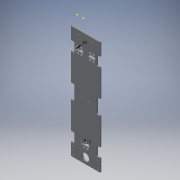
# Autodesk Inventor part: XCartFloor
Saved by Autodesk Inventor 2019 (Build 230136000, 136)
## iProperties
Created: 2019-08-19
Part Number: XCartFloor
Material: Generic
Document SubType Name: Modeling
Designer: Bruno
Density: 1 g/cm^3
Appearance: Default
Author: Bruno
Autodesk Inventor part; units mm, degrees
ref_plane "YZ Plane" through (0, 0, 0) normal (1, 0, 0) x (0, 1, 0)
ref_plane "XZ Plane" through (0, 0, 0) normal (0, 1, 0) x (-1, 0, 0)
ref_plane "XY Plane" through (0, 0, 0) normal (0, 0, 1) x (1, 0, 0)
sketch "Sketch1" plane through (0, 0, 0) normal (0, 0, 1) x (1, 0, 0)
  line L0 (100.0979, -38.5222) -> (0.0979, -38.5222)
  line L1 (0.0979, -426.5222) -> (100.0979, -426.5222)
  line L2 (82.7645, -93.1222) -> (58.7645, -93.1222)
  line L3 (58.7645, -93.1222) -> (58.7645, -101.9222)
  line L4 (58.7645, -101.9222) -> (82.7645, -101.9222)
  line L5 (82.7645, -101.9222) -> (82.7645, -93.1222)
  line L6 (41.4312, -93.1222) -> (17.4312, -93.1222)
  line L7 (17.4312, -93.1222) -> (17.4312, -101.9222)
  line L8 (17.4312, -101.9222) -> (41.4312, -101.9222)
  line L9 (41.4312, -101.9222) -> (41.4312, -93.1222)
  line L10 (38.0979, -363.1222) -> (62.0979, -363.1222)
  line L11 (62.0979, -363.1222) -> (62.0979, -371.9222)
  line L12 (62.0979, -371.9222) -> (38.0979, -371.9222)
  line L13 (38.0979, -371.9222) -> (38.0979, -363.1222)
  line L14 (173.8639, -93.5222) -> (-221.1361, -93.5222)
  line L15 (173.8639, -101.5222) -> (-221.1361, -101.5222)
  line L16 (173.8639, -371.5222) -> (-221.1361, -371.5222)
  line L17 (173.8639, -363.5222) -> (-221.1361, -363.5222)
  line L18 (34.8712, -93.1222) -> (34.8712, -93.5222) construction
  line L19 (34.8712, -101.5222) -> (34.8712, -101.9222) construction
  line L20 (58.7645, -93.1222) -> (41.4312, -93.1222) construction
  line L21 (10.9151, -363.1222) -> (10.9151, -363.5222) construction
  line L22 (10.9151, -371.5222) -> (10.9151, -371.9222) construction
  line L23 (38.0979, -363.1222) -> (12.0979, -363.1222) construction
  line L24 (62.0979, -363.1222) -> (88.0979, -363.1222) construction
  line L25 (0, 0) -> (0, -9.7735) construction
  circle A0 centre (65.5979, -390.5222) radius 1.625
  circle A1 centre (65.5979, -421.5222) radius 1.625
  circle A2 centre (34.5979, -421.5222) radius 1.625
  circle A3 centre (34.5979, -390.5222) radius 1.625
  line L26 (65.5979, -390.5222) -> (34.5979, -390.5222) construction
  line L27 (34.5979, -390.5222) -> (34.5979, -421.5222) construction
  line L28 (34.5979, -421.5222) -> (65.5979, -421.5222) construction
  line L29 (65.5979, -421.5222) -> (65.5979, -390.5222) construction
  circle A4 centre (50.0979, -406.0222) radius 12.5
  line L30 (50.0979, -390.5222) -> (50.0979, -406.0222) construction
  line L31 (50.0979, -406.0222) -> (65.5979, -406.0222) construction
  line L32 (72.2645, -85.1222) -> (80.2645, -85.1222)
  line L33 (80.2645, -85.1222) -> (80.2645, -89.1222)
  line L34 (80.2645, -89.1222) -> (72.2645, -89.1222)
  line L35 (72.2645, -89.1222) -> (72.2645, -85.1222)
  line L36 (80.2645, -89.1222) -> (82.7645, -89.1222) construction
  line L37 (82.7645, -89.1222) -> (82.7645, -93.1222) construction
  line L38 (69.2645, -85.1222) -> (61.2645, -85.1222)
  line L39 (61.2645, -85.1222) -> (61.2645, -89.1222)
  line L40 (61.2645, -89.1222) -> (69.2645, -89.1222)
  line L41 (69.2645, -89.1222) -> (69.2645, -85.1222)
  line L42 (58.7645, -93.1222) -> (58.7645, -89.1222) construction
  line L43 (58.7645, -89.1222) -> (61.2645, -89.1222) construction
  line L44 (72.2645, -105.9222) -> (80.2645, -105.9222)
  line L45 (80.2645, -105.9222) -> (80.2645, -109.9222)
  line L46 (80.2645, -109.9222) -> (72.2645, -109.9222)
  line L47 (72.2645, -109.9222) -> (72.2645, -105.9222)
  line L48 (80.2645, -105.9222) -> (80.2645, -101.9222) construction
  line L49 (69.2645, -105.9222) -> (61.2645, -105.9222)
  line L50 (61.2645, -105.9222) -> (61.2645, -109.9222)
  line L51 (61.2645, -109.9222) -> (69.2645, -109.9222)
  line L52 (69.2645, -109.9222) -> (69.2645, -105.9222)
  line L53 (38.9312, -85.1222) -> (30.9312, -85.1222)
  line L54 (30.9312, -85.1222) -> (30.9312, -89.1222)
  line L55 (30.9312, -89.1222) -> (38.9312, -89.1222)
  line L56 (38.9312, -89.1222) -> (38.9312, -85.1222)
  line L57 (27.9312, -85.1222) -> (19.9312, -85.1222)
  line L58 (19.9312, -85.1222) -> (19.9312, -89.1222)
  line L59 (19.9312, -89.1222) -> (27.9312, -89.1222)
  line L60 (27.9312, -89.1222) -> (27.9312, -85.1222)
  line L61 (30.9312, -105.9222) -> (38.9312, -105.9222)
  line L62 (38.9312, -105.9222) -> (38.9312, -109.9222)
  line L63 (38.9312, -109.9222) -> (30.9312, -109.9222)
  line L64 (30.9312, -109.9222) -> (30.9312, -105.9222)
  line L65 (27.9312, -105.9222) -> (19.9312, -105.9222)
  line L66 (19.9312, -105.9222) -> (19.9312, -109.9222)
  line L67 (19.9312, -109.9222) -> (27.9312, -109.9222)
  line L68 (27.9312, -109.9222) -> (27.9312, -105.9222)
  line L69 (41.4312, -93.1222) -> (41.4312, -89.1222) construction
  line L70 (41.4312, -89.1222) -> (38.9312, -89.1222) construction
  line L71 (17.4312, -93.1222) -> (17.4312, -89.1222) construction
  line L72 (17.4312, -89.1222) -> (19.9312, -89.1222) construction
  line L73 (51.5979, -355.1222) -> (59.5979, -355.1222)
  line L74 (59.5979, -355.1222) -> (59.5979, -359.1222)
  line L75 (59.5979, -359.1222) -> (51.5979, -359.1222)
  line L76 (51.5979, -359.1222) -> (51.5979, -355.1222)
  line L77 (48.5979, -355.1222) -> (40.5979, -355.1222)
  line L78 (40.5979, -355.1222) -> (40.5979, -359.1222)
  line L79 (40.5979, -359.1222) -> (48.5979, -359.1222)
  line L80 (48.5979, -359.1222) -> (48.5979, -355.1222)
  line L81 (51.5979, -375.9222) -> (59.5979, -375.9222)
  line L82 (59.5979, -375.9222) -> (59.5979, -379.9222)
  line L83 (59.5979, -379.9222) -> (51.5979, -379.9222)
  line L84 (51.5979, -379.9222) -> (51.5979, -375.9222)
  line L85 (48.5979, -375.9222) -> (40.5979, -375.9222)
  line L86 (40.5979, -375.9222) -> (40.5979, -379.9222)
  line L87 (40.5979, -379.9222) -> (48.5979, -379.9222)
  line L88 (48.5979, -379.9222) -> (48.5979, -375.9222)
  line L89 (59.5979, -359.1222) -> (62.0979, -359.1222) construction
  line L90 (62.0979, -359.1222) -> (62.0979, -363.1222) construction
  line L91 (38.0979, -363.1222) -> (38.0979, -359.1222) construction
  line L92 (38.0979, -359.1222) -> (40.5979, -359.1222) construction
  line L93 (59.5979, -375.9222) -> (59.5979, -371.9222) construction
  circle A5 centre (73.5979, -50.5222) radius 2.125
  circle A6 centre (26.5979, -50.5222) radius 2.125
  line L94 (73.5979, -50.5222) -> (100.0979, -50.5222) construction
  line L95 (26.5979, -50.5222) -> (0.0979, -50.5222) construction
  line L96 (96.5979, -57.5222) -> (88.5979, -57.5222) projected
  line L97 (11.5979, -57.5222) -> (3.5979, -57.5222) projected
  line L98 (8.0979, -43.5222) -> (8.0979, -57.5222) projected
  line L99 (7.0979, -57.5222) -> (7.0979, -43.5222) projected
  line L100 (93.0979, -43.5222) -> (93.0979, -57.5222) projected
  line L101 (92.0979, -57.5222) -> (92.0979, -43.5222) projected
  line L102 (7.5979, -57.5222) -> (7.5979, -426.5222) construction
  line L103 (92.5979, -57.5222) -> (92.5979, -426.5222) construction
  circle A7 centre (92.5979, -419.5222) radius 2.125
  circle A8 centre (92.5979, -392.5222) radius 2.125
  circle A9 centre (7.5979, -419.5222) radius 2.125
  circle A10 centre (7.5979, -392.5222) radius 2.125
  line L104 (92.5979, -419.5222) -> (7.5979, -419.5222) construction
  line L105 (92.5979, -392.5222) -> (7.5979, -392.5222) construction
  line L106 (100.0979, -38.5222) -> (100.0979, -81.5222)
  line L107 (100.0979, -81.5222) -> (88.0979, -81.5222)
  line L108 (88.0979, -81.5222) -> (88.0979, -113.5222)
  line L109 (88.0979, -113.5222) -> (100.0979, -113.5222)
  line L110 (100.0979, -351.5222) -> (88.0979, -351.5222)
  line L111 (88.0979, -351.5222) -> (88.0979, -383.5222)
  line L112 (88.0979, -383.5222) -> (100.0979, -383.5222)
  line L113 (100.0979, -383.5222) -> (100.0979, -426.5222)
  line L114 (100.0979, -81.5222) -> (100.0979, -93.5222) construction
  line L115 (100.0979, -101.5222) -> (100.0979, -113.5222) construction
  line L116 (0.0979, -38.5222) -> (0.0979, -81.5222)
  line L117 (0.0979, -81.5222) -> (12.0979, -81.5222)
  line L118 (12.0979, -81.5222) -> (12.0979, -113.5222)
  line L119 (12.0979, -113.5222) -> (0.0979, -113.5222)
  line L120 (0.0979, -351.5222) -> (12.0979, -351.5222)
  line L121 (12.0979, -351.5222) -> (12.0979, -383.5222)
  line L122 (12.0979, -383.5222) -> (0.0979, -383.5222)
  line L123 (0.0979, -383.5222) -> (0.0979, -426.5222)
  line L124 (98.1469, -351.5222) -> (98.1469, -363.5222) construction
  line L125 (98.1469, -383.5222) -> (98.1469, -371.5222) construction
  line L126 (17.4312, -93.1222) -> (12.0979, -93.1222) construction
  line L127 (82.7645, -93.1222) -> (88.0979, -93.1222) construction
  line L128 (82.7645, -97.5222) -> (100.0979, -97.5222) construction
  line L129 (58.7645, -97.5222) -> (41.4312, -97.5222) construction
  line L130 (17.4312, -97.5222) -> (0.0979, -97.5222) construction
  line L131 (38.0979, -367.5222) -> (0.0979, -367.5222) construction
  line L132 (62.0979, -367.5222) -> (100.0979, -367.5222) construction
  line L133 (100.0979, -113.5222) -> (100.0979, -207.5222)
  line L134 (100.0979, -207.5222) -> (88.0979, -207.5222)
  line L135 (88.0979, -207.5222) -> (88.0979, -257.5222)
  line L136 (88.0979, -257.5222) -> (100.0979, -257.5222)
  line L137 (100.0979, -257.5222) -> (100.0979, -351.5222)
  line L138 (0.0979, -113.5222) -> (0.0979, -207.5222)
  line L139 (0.0979, -207.5222) -> (12.0979, -207.5222)
  line L140 (12.0979, -207.5222) -> (12.0979, -257.5222)
  line L141 (12.0979, -257.5222) -> (0.0979, -257.5222)
  line L142 (0.0979, -257.5222) -> (0.0979, -351.5222)
  line L143 (34.5979, -390.5222) -> (0.0979, -390.5222) construction
  line L144 (65.5979, -390.5222) -> (100.0979, -390.5222) construction
  circle A11 centre (40.0979, -232.5222) radius 2.125
  circle A12 centre (60.0979, -232.5222) radius 2.125
  line L145 (40.0979, -232.5222) -> (60.0979, -232.5222) construction
  line L146 (40.0979, -232.5222) -> (12.0979, -232.5222) construction
  line L147 (60.0979, -232.5222) -> (88.0979, -232.5222) construction
  dimension "d1" = 24
  dimension "d2" = 8.8
  dimension "d3" = 100
  dimension "d9" = 55
  dimension "d10" = 55
  dimension "d11" = 3.25
  dimension "d12" = 31
  dimension "d13" = 5
  dimension "d14" = 25
  dimension "d15" = 4
  dimension "d16" = 8
  dimension "d17" = 4
  dimension "d18" = 2.5
  dimension "d19" = 4.25
  dimension "d20" = 4.25
  dimension "d21" = 47
  dimension "d22" = 12
  dimension "d23" = 4.25
  dimension "d24" = 4.25
  dimension "d25" = 27
  dimension "d26" = 7
  dimension "d27" = 4.25
  dimension "d28" = 4.25
  dimension "d29" = 32
  dimension "d30" = 12
  dimension "d31" = 50
  dimension "d32" = 4.25
  dimension "d33" = 4.25
  dimension "d34" = 20
  dimension "d35" = 25
  constraints: 284 end point, 64 point on line, 48 perpendicular, 47 equal length, 34 parallel, 31 horizontal, 18 collinear, 15 vertical, 13 centre point, 12 midpoint, 3 equal radius, 8 other
  measures "d1" distance of L3.end L4.end
  measures "d2" distance of L2.end L3.end
  measures "d3" distance of L0.start L0.end
  measures "d9" distance between parallel lines of L0 L14
  measures "d10" distance between parallel lines of L1 L16
  measures "d11" diameter of A0
  measures "d12" distance of L28.end L26.start
  measures "d13" distance between parallel lines of L1 L28
  measures "d14" diameter of A4
  measures "d15" distance of L32.end L33.end
  measures "d16" distance of L32.start L32.end
  measures "d17" distance of L36.end L2.start
  measures "d18" distance of L33.end L36.end
  measures "d19" diameter of A5
  measures "d20" diameter of A6
  measures "d21" distance of L95.start L94.start
  measures "d22" distance between parallel lines of L0 L94
  measures "d23" diameter of A7
  measures "d24" diameter of A8
  measures "d25" distance of L104.start L105.start
  measures "d26" distance from line of L1 L104.start
  measures "d27" diameter of A9
  measures "d28" diameter of A10
  measures "d29" distance of L107.end L108.end
  measures "d30" distance of L108.end L109.end
  measures "d31" distance of L134.end L135.end
  measures "d32" diameter of A11
  measures "d33" diameter of A12
  measures "d34" distance of L145.start L145.end
  measures "d35" distance between parallel lines of L141 L146
extrude "Extrusion1" add sketch "Sketch1" along normal blind 5 contours L106 L107 L108 L14 L5 L2 L3 L9 L6 L7 L118 L117 L116 L0 | L108 L15 L5 L14 | L14 L7 L15 L118 | L108 L109 L133 L134 L135 L136 L137 L110 L111 L17 L11 L10 L13 L121 L120 L142 L141 L140 L139 L138 L119 L118 L15 L7 L8 L9 L3 L4 L5 | L3 L15 L9 L14 | L111 L16 L11 L17 | L17 L13 L16 L121 | L111 L112 L113 L1 L123 L122 L121 L16 L13 L12 L11
sketch "Sketch2" plane through (17.4312, -101.9222, 0) normal (1, 0, 0) x (0, 0, -1)
  circle A0 centre (6.0737, 4.4) radius 7.5
  point P0 (0, 101.9222)
  point P1 (0, 8.8)
  point P2 (0, 0)
  dimension "d6" = 15
  constraints: 2 point on circle, 1 centre point
  measures "d6" diameter of A0
sketch "Sketch3" plane through (38.0979, -371.9222, 0) normal (1, 0, 0) x (0, 0, -1)
  circle A0 centre (6.0737, 4.4) radius 7.5
  point P0 (0, 371.9222)
  point P1 (0, 8.8)
  point P2 (0, 0)
  dimension "d8" = 15
  constraints: 2 point on circle, 1 centre point
  measures "d8" diameter of A0
body "Solid1"
